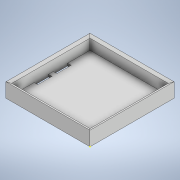
# Autodesk Inventor part: led-compartment-2
Saved by Autodesk Inventor 2021 (Build 250183000, 183)
## iProperties
Created: 2021-01-17
Part Number: led-compartment-2
Material: Generic
Document SubType Name: Modeling
Designer: Luke Kamols
Density: 1 g/cm^3
Appearance: Default
Author: Luke Kamols
Autodesk Inventor part; units mm, degrees
ref_plane "YZ Plane" through (0, 0, 0) normal (1, 0, 0) x (0, 1, 0)
ref_plane "XZ Plane" through (0, 0, 0) normal (0, 1, 0) x (-1, 0, 0)
ref_plane "XY Plane" through (0, 0, 0) normal (0, 0, 1) x (1, 0, 0)
sketch "Sketch1" plane through (0, 0, 0) normal (0, 1, 0) x (-1, 0, 0)
  point P0 (0, 0)
sketch "Sketch2" plane through (0, 0, 0) normal (0, 1, 0) x (-1, 0, 0)
  line L0 (0, 0) -> (35.2, 0)
  line L1 (35.2, 0) -> (35.2, -35.2)
  line L2 (35.2, -35.2) -> (0, -35.2)
  line L3 (0, -35.2) -> (0, 0)
  dimension "d0" = 35.2
  dimension "d1" = 35.2
  constraints: 8 end point, 2 parallel, 1 horizontal, 1 perpendicular
  measures "d0" distance of L1.end L2.end
  measures "d1" distance of L0.end L1.end
extrude "Extrusion1" add sketch "Sketch2" along normal blind 1
sketch "Sketch3" plane through (0, 1, 0) normal (0, 1, 0) x (1, 0, 0)
  line L0 (0, 35.2) -> (-35.2, 35.2) projected
  line L1 (-35.2, 35.2) -> (-35.2, 0) projected
  line L2 (-35.2, 0) -> (0, 0) projected
  line L3 (0, 0) -> (0, 35.2) projected
  line L4 (-35.2, 0) -> (0, 0) projected
  line L5 (0, 0) -> (-1.2, 0)
  line L6 (-1.2, 0) -> (-1.2, 1.2)
  line L7 (-1.2, 1.2) -> (-34, 1.2)
  line L8 (-34, 1.2) -> (-34, 34)
  line L9 (-34, 34) -> (-1.2, 34)
  line L10 (-1.2, 34) -> (-1.2, 1.2)
  dimension "d4" = 1.2
  dimension "d5" = 1.2
  dimension "d6" = 32.8
  dimension "d7" = 32.8
  constraints: 12 end point, 2 parallel, 2 perpendicular, 1 horizontal, 1 point on line
  measures "d4" distance of L4.end L5.end
  measures "d5" distance of L5.end L6.end
  measures "d6" distance of L8.end L9.end
  measures "d7" distance of L7.end L8.end
extrude "Extrusion2" add sketch "Sketch3" along normal blind 5
sketch "Sketch4" plane through (0, 1, 0) normal (0, 1, 0) x (1, 0, 0)
  line L0 (-1.2, 1.2) -> (-1.2, 34) projected
  line L1 (-1.2, 34) -> (-34, 34) projected
  line L2 (-34, 34) -> (-34, 1.2) projected
  line L3 (-34, 1.2) -> (-1.2, 1.2) projected
  line L4 (-1.2, 1.2) -> (-1.2, 34) projected
  line L5 (-1.2, 17.6) -> (-34, 17.6)
  line L6 (-34, 34) -> (-1.2, 34) projected
  line L7 (-17.6, 34) -> (-17.6, 1.2)
  line L8 (-17.6, 17.6) -> (-17.6, 18.6)
  line L9 (-34, 17.6) -> (-34, 17.6)
  line L10 (-34, 1.2) -> (-34, 34) projected
  line L11 (-34, 17.6) -> (-32.5, 17.6)
  line L12 (-1.2, 17.6) -> (-1.2, 18.6)
  line L13 (-1.2, 18.6) -> (-2.7, 18.6)
  line L14 (-2.7, 18.6) -> (-2.7, 24.6)
  line L15 (-2.7, 24.6) -> (-1.2, 24.6)
  line L16 (-1.2, 17.6) -> (-1.2, 15.6)
  line L17 (-1.2, 17.6) -> (-1.2, 16.6)
  line L18 (-1.2, 34) -> (-1.2, 1.2) projected
  line L19 (-1.2, 16.6) -> (-2.7, 16.6)
  line L20 (-2.7, 16.6) -> (-2.7, 10.6)
  line L21 (-2.7, 10.6) -> (-1.2, 10.6)
  line L22 (-34, 17.6) -> (-34, 18.6)
  line L23 (-34, 1.2) -> (-34, 34) projected
  line L24 (-34, 18.6) -> (-32.5, 18.6)
  line L25 (-32.5, 18.6) -> (-32.5, 24.6)
  line L26 (-32.5, 24.6) -> (-34, 24.6)
  line L27 (-34, 17.6) -> (-34, 16.6)
  line L28 (-34, 16.6) -> (-32.5, 16.6)
  line L29 (-32.5, 16.6) -> (-32.5, 10.6)
  line L30 (-32.5, 10.6) -> (-34, 10.6)
  point P0 (0, 0)
  point P1 (-34, 23.6)
  dimension "d13" = 1
  dimension "d19" = 1.5
  dimension "d20" = 6
  dimension "d49" = 6
  constraints: 44 end point, 11 point on line, 10 perpendicular, 6 midpoint, 3 horizontal
  measures "d13" distance of L8.start L8.end
  measures "d19" distance of L12.end L13.end
  measures "d20" distance of L13.end L14.end
  measures "d49" distance of L19.end L20.end
extrude "Extrusion3" cut sketch "Sketch4" against normal blind 4 contours L21 L20 L19 L0 | L2 L28 L29 L30 | L13 L14 L15 L0 | L2 L26 L25 L24
chamfer "Chamfer3" distance 1.2 distance2 0.6 1 edges at (-1.2, 6, -17.6) measured on face at (-34.8, 6, -23.0667)
chamfer "Chamfer4" distance 1.2 distance2 0.6 1 edges at (-17.6, 6, -1.2) measured on face at (-34.8, 6, -23.0667)
chamfer "Chamfer5" distance 1.2 distance2 0.6 1 edges at (-17.6, 6, -34) measured on face at (-34.8, 6, -23.0667)
chamfer "Chamfer6" distance 1.2 distance2 0.6 1 edges at (-34, 6, -17.6) measured on face at (-34.8, 6, -23.0667)
body "Solid1"
